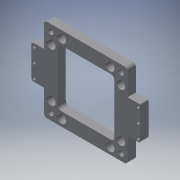
# Autodesk Inventor part: 20_IM_LED_holder
Saved by Autodesk Inventor 2019 (Build 230136000, 136)
## iProperties
Created: 2020-10-28
Part Number: 20_IM_LED_holder
Material: Generic
Document SubType Name: Modeling
Designer: wanghaoran
Density: 1 g/cm^3
Appearance: Default
Author: wanghaoran
Autodesk Inventor part; units mm, degrees
ref_plane "YZ Plane" through (0, 0, 0) normal (1, 0, 0) x (0, 1, 0)
ref_plane "XZ Plane" through (0, 0, 0) normal (0, 1, 0) x (-1, 0, 0)
sketch "Sketch1" plane through (0, 0, 0) normal (0, 0, 1) x (1, 0, 0)
  line L0 (-25, 25) -> (25, 25)
  line L1 (25, 25) -> (25, -25)
  line L2 (25, -25) -> (-25, -25)
  line L3 (-25, -25) -> (-25, 25)
  line L4 (-25, 25) -> (25, -25) construction
  line L5 (25, 25) -> (-25, -25) construction
  circle A0 centre (0, 0) radius 2.5
  circle A1 centre (-20.8, -14.5) radius 2.65
  circle A2 centre (-14.5, -20.8) radius 2.65
  circle A3 centre (-20.8, 14.5) radius 2.65
  circle A4 centre (20.8, -14.5) radius 2.65
  circle A5 centre (20.8, 14.5) radius 2.65
  circle A6 centre (-14.5, 20.8) radius 2.65
  circle A7 centre (14.5, -20.8) radius 2.65
  circle A8 centre (14.5, 20.8) radius 2.65
  dimension "d0" = 50
  dimension "d1" = 50
  dimension "d2" = 5
  dimension "d5" = 5.3
  dimension "d6" = 4.2
  dimension "d8" = 10.5
  dimension "d11" = 29
  dimension "d14" = 41.6
  constraints: 12 end point, 9 centre point, 4 symmetric about line, 2 horizontal, 2 midpoint, 2 parallel, 1 coincident, 1 perpendicular, 1 vertical, 10 other
  measures "d0" distance of L1.end L2.end
  measures "d1" distance of L0.end L1.end
  measures "d2" diameter of A0
  measures "d5" diameter of A1
  measures "d6" distance from line of A1.centre L3
  measures "d8" distance from line of L2 A1.centre
  measures "d11" distance of A1.centre A3.centre
  measures "d14" distance of A1.centre A4.centre
extrude "Extrusion1" add sketch "Sketch1" along normal blind 4
fillet "Fillet1" radius 2 4 edges at (-25, 25, 2) (25, 25, 2) (-25, -25, 2) (25, -25, 2)
sketch "Sketch2" plane through (0, 0, 4) normal (0, 0, 1) x (1, 0, 0)
  arc A0 (23, -25) -> (25, -23) centre (23, -23) ccw projected
  line L0 (25, -23) -> (25, 23) projected
  arc A1 (25, 23) -> (23, 25) centre (23, 23) ccw projected
  line L1 (23, 25) -> (-23, 25) projected
  arc A2 (-23, 25) -> (-25, 23) centre (-23, 23) ccw projected
  line L2 (-25, 23) -> (-25, -23) projected
  arc A3 (-25, -23) -> (-23, -25) centre (-23, -23) ccw projected
  line L3 (-23, -25) -> (23, -25) projected
  circle A4 centre (14.5, 20.8) radius 2.65 projected
  circle A5 centre (-14.5, 20.8) radius 2.65 projected
  circle A6 centre (14.5, -20.8) radius 2.65 projected
  circle A7 centre (20.8, 14.5) radius 2.65 projected
  circle A8 centre (20.8, -14.5) radius 2.65 projected
  circle A9 centre (-20.8, 14.5) radius 2.65 projected
  circle A10 centre (-14.5, -20.8) radius 2.65 projected
  circle A11 centre (-20.8, -14.5) radius 2.65 projected
  circle A12 centre (0, 0) radius 2.5 projected
  line L4 (21, -21) -> (-21, -21)
  line L5 (-21, -21) -> (-21, 21)
  line L6 (-21, 21) -> (21, 21)
  line L7 (21, 21) -> (21, -21)
  line L8 (21, -21) -> (-21, 21) construction
  line L9 (-21, -21) -> (21, 21) construction
  circle A13 centre (-28.6, 21.06) radius 1.55 projected
  dimension "d18" = 42
  dimension "d19" = 42
  constraints: 12 end point, 2 midpoint, 2 parallel, 1 horizontal, 1 perpendicular
  measures "d18" distance of L5.end L6.end
  measures "d19" distance of L4.end L5.end
hole "Hole1" at (-21, 21, 4) at (21, 21, 4) at (21, -21, 4) at (-21, -21, 4) direction (0, 0, -1) diameter 3.3 end through all both
sketch "Sketch4" plane through (0, 0, 4) normal (0, 0, 1) x (1, 0, 0)
  circle A0 centre (21, -21) radius 1.65 construction
  circle A1 centre (-21, 21) radius 1.65 construction
  circle A2 centre (21, 21) radius 1.65 construction
  circle A3 centre (-21, -21) radius 1.65 construction
  arc A4 (23, -25) -> (25, -23) centre (23, -23) ccw projected
  line L0 (25, -23) -> (25, 23) projected
  arc A5 (25, 23) -> (23, 25) centre (23, 23) ccw projected
  line L1 (23, 25) -> (-23, 25) projected
  arc A6 (-23, 25) -> (-25, 23) centre (-23, 23) ccw projected
  line L2 (-25, 23) -> (-25, -23) projected
  arc A7 (-25, -23) -> (-23, -25) centre (-23, -23) ccw projected
  line L3 (-23, -25) -> (23, -25) projected
  circle A8 centre (14.5, 20.8) radius 2.65 construction
  circle A9 centre (-14.5, 20.8) radius 2.65 construction
  circle A10 centre (14.5, -20.8) radius 2.65 construction
  circle A11 centre (20.8, 14.5) radius 2.65 construction
  circle A12 centre (20.8, -14.5) radius 2.65 construction
  circle A13 centre (-20.8, 14.5) radius 2.65 construction
  circle A14 centre (-14.5, -20.8) radius 2.65 construction
  circle A15 centre (-20.8, -14.5) radius 2.65 construction
  circle A16 centre (0, 0) radius 2.5 construction
  line L4 (17, -15) -> (17, 15)
  line L5 (15, 17) -> (-15, 17)
  line L6 (-17, 15) -> (-17, -15)
  line L7 (-15, -17) -> (15, -17)
  arc A17 (15, -17) -> (17, -15) centre (15, -15) ccw
  arc A18 (-17, -15) -> (-15, -17) centre (-15, -15) ccw
  arc A19 (-15, 17) -> (-17, 15) centre (-15, 15) ccw
  arc A20 (17, 15) -> (15, 17) centre (15, 15) ccw
  dimension "d34" = 8
  dimension "d35" = 2
  constraints: 8 end point, 8 point on circle, 8 tangent, 4 centre point, 3 equal radius, 3 other
  measures "d34" distance between parallel lines of L3 L7
  measures "d35" radius of A17
extrude "Extrusion2" cut sketch "Sketch4" against normal through all contours A17 L7 A18 L6 A19 L5 A20 L4
sketch "Sketch5" plane through (0, 0, 4) normal (0, 0, 1) x (1, 0, 0)
  arc A0 (17, 15) -> (15, 17) centre (15, 15) ccw construction
  line L0 (17, 15) -> (17, -15) construction
  arc A1 (15, -17) -> (17, -15) centre (15, -15) ccw construction
  line L1 (15, -17) -> (-15, -17) construction
  arc A2 (-17, -15) -> (-15, -17) centre (-15, -15) ccw construction
  line L2 (-17, -15) -> (-17, 15) construction
  arc A3 (-15, 17) -> (-17, 15) centre (-15, 15) ccw construction
  line L3 (-15, 17) -> (15, 17) construction
  circle A4 centre (21, -21) radius 1.65 construction
  circle A5 centre (-21, 21) radius 1.65 construction
  circle A6 centre (21, 21) radius 1.65 construction
  circle A7 centre (-21, -21) radius 1.65 construction
  arc A8 (23, -25) -> (25, -23) centre (23, -23) ccw construction
  line L4 (25, -23) -> (25, 23) construction
  arc A9 (25, 23) -> (23, 25) centre (23, 23) ccw construction
  line L5 (23, 25) -> (-23, 25) construction
  arc A10 (-23, 25) -> (-25, 23) centre (-23, 23) ccw construction
  line L6 (-25, 23) -> (-25, -23) construction
  arc A11 (-25, -23) -> (-23, -25) centre (-23, -23) ccw construction
  line L7 (-23, -25) -> (23, -25) construction
  circle A12 centre (14.5, 20.8) radius 2.65 construction
  circle A13 centre (-14.5, 20.8) radius 2.65 construction
  circle A14 centre (14.5, -20.8) radius 2.65 construction
  circle A15 centre (20.8, 14.5) radius 2.65 construction
  circle A16 centre (20.8, -14.5) radius 2.65 construction
  circle A17 centre (-20.8, 14.5) radius 2.65 construction
  circle A18 centre (-14.5, -20.8) radius 2.65 construction
  circle A19 centre (-20.8, -14.5) radius 2.65 construction
  circle A20 centre (31.1, -8.2) radius 1
  circle A21 centre (31.1, 0) radius 1
  circle A22 centre (31.1, 8.2) radius 1
  line L8 (25, 23) -> (25, -23) projected
  line L9 (33, -10) -> (25, -10)
  line L10 (25, -10) -> (25, 10)
  line L11 (25, 10) -> (33, 10)
  line L12 (0, 45.5) -> (0, -45.5) construction
  arc A23 (33, -10) -> (34, -9.0093) centre (33, -9) ccw
  arc A24 (34, 9) -> (33, 10) centre (33, 9) ccw
  line L13 (45.5, 0) -> (-45.5, 0) construction
  line L14 (-34, -9.0093) -> (-34, 9) construction
  circle A25 centre (-31.1, -8.2) radius 1
  circle A26 centre (-31.1, 0) radius 1
  circle A27 centre (-31.1, 8.2) radius 1
  line L15 (-33, -10) -> (-25, -10)
  line L16 (-25, -10) -> (-25, 10)
  line L17 (-25, 10) -> (-33, 10)
  line L18 (-34, 9) -> (-34, -9.0093)
  arc A28 (-34, -9.0093) -> (-33, -10) centre (-33, -9) ccw
  arc A29 (-33, 10) -> (-34, 9) centre (-33, 9) ccw
  line L19 (34, 9) -> (34, -9.0093)
  point P0 (0, 0)
  point P1 (34, -10)
  point P2 (32.5, 10)
  point P3 (-34, -10)
  point P4 (-32.5, 10)
  dimension "d38" = 20
  dimension "d39" = 1
  dimension "d40" = 1
  dimension "d43" = 9
  constraints: 22 end point, 13 symmetric about line, 10 centre point, 8 point on circle, 6 point on line, 2 horizontal, 2 tangent, 2 vertical, 1 parallel, 1 perpendicular, 16 other
  measures "d38" distance between parallel lines of L11 L9
  measures "d39" radius of A23
  measures "d40" radius of A24
  measures "d43" distance between parallel lines of L19 L4
ref_plane "Work Plane1" through (-32.5, -32.5, -1) normal (0, 0, -1) x (0, 1, 0)
extrude "Extrusion3" add sketch "Sketch5" against normal up to surface (4 mm away)
body "Solid1"
